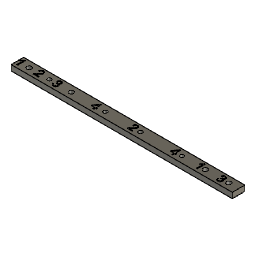
Base Board Tester v1 (Autodesk Fusion 360 design; units mm, degrees)
Autodesk Fusion 360 part; units mm, degrees
sketch "Sketch1" plane through (0, 0, 0) normal (0, 0, 1) x (1, 0, 0)
  line L0 (-51.9584, -20.427) -> (88.8166, -20.427)
  line L1 (88.8166, -20.427) -> (88.8166, -28.427)
  line L2 (88.8166, -28.427) -> (-51.9584, -28.427)
  line L3 (-51.9584, -28.427) -> (-51.9584, -20.427)
  circle A0 centre (-17.6214, -24.427) radius 1.5
  circle A1 centre (82.5086, -24.427) radius 1.5
  circle A2 centre (-44.4942, -24.427) radius 1.5
  circle A3 centre (67.7058, -24.427) radius 1.5
  circle A4 centre (4, -24.427) radius 1.25
  circle A5 centre (52.78, -24.427) radius 1.25
  circle A6 centre (-31.6334, -24.427) radius 1.25
  circle A7 centre (26.3666, -24.427) radius 1.25
  line L4 (-49.5707, -26.5817) -> (-50.1846, -26.5817)
  line L5 (-50.1846, -26.5817) -> (-50.1846, -22.6697)
  spline S0 degree 2 poles (-50.1846, -22.6697) (-50.4063, -22.8811) (-50.7679, -23.0926) knots 0 0 0 1 1 1
  spline S1 degree 2 poles (-50.7679, -23.0926) (-51.126, -23.304) (-51.4125, -23.4098) knots 0 0 0 1 1 1
  line L6 (-51.4125, -23.4098) -> (-51.4125, -22.8163)
  spline S2 degree 2 poles (-51.4125, -22.8163) (-50.8975, -22.5742) (-50.5121, -22.2297) knots 0 0 0 1 1 1
  spline S3 degree 2 poles (-50.5121, -22.2297) (-50.1267, -21.8852) (-49.9664, -21.5612) knots 0 0 0 1 1 1
  line L7 (-49.9664, -21.5612) -> (-49.5707, -21.5612)
  line L8 (-49.5707, -21.5612) -> (-49.5707, -26.5817)
  line L9 (-36.5983, -26.0261) -> (-36.5983, -26.6161)
  line L10 (-36.5983, -26.6161) -> (-39.9033, -26.6161)
  spline S4 degree 2 poles (-39.9033, -26.6161) (-39.9101, -26.3944) (-39.8316, -26.1898) knots 0 0 0 1 1 1
  spline S5 degree 2 poles (-39.8316, -26.1898) (-39.7054, -25.8521) (-39.4292, -25.5247) knots 0 0 0 1 1 1
  spline S6 degree 2 poles (-39.4292, -25.5247) (-39.1495, -25.1973) (-38.6243, -24.7675) knots 0 0 0 1 1 1
  spline S7 degree 2 poles (-38.6243, -24.7675) (-37.8091, -24.0991) (-37.5226, -23.7102) knots 0 0 0 1 1 1
  spline S8 degree 2 poles (-37.5226, -23.7102) (-37.2361, -23.318) (-37.2361, -22.9701) knots 0 0 0 1 1 1
  spline S9 degree 2 poles (-37.2361, -22.9701) (-37.2361, -22.6052) (-37.4988, -22.3562) knots 0 0 0 1 1 1
  spline S10 degree 2 poles (-37.4988, -22.3562) (-37.758, -22.1038) (-38.1775, -22.1038) knots 0 0 0 1 1 1
  spline S11 degree 2 poles (-38.1775, -22.1038) (-38.6209, -22.1038) (-38.8869, -22.3699) knots 0 0 0 1 1 1
  spline S12 degree 2 poles (-38.8869, -22.3699) (-39.1529, -22.6359) (-39.1563, -23.1066) knots 0 0 0 1 1 1
  line L11 (-39.1563, -23.1066) -> (-39.7873, -23.0418)
  spline S13 degree 2 poles (-39.7873, -23.0418) (-39.7225, -22.3358) (-39.2996, -21.9674) knots 0 0 0 1 1 1
  spline S14 degree 2 poles (-39.2996, -21.9674) (-38.8767, -21.5957) (-38.1638, -21.5957) knots 0 0 0 1 1 1
  spline S15 degree 2 poles (-38.1638, -21.5957) (-37.4442, -21.5957) (-37.0247, -21.9947) knots 0 0 0 1 1 1
  spline S16 degree 2 poles (-37.0247, -21.9947) (-36.6052, -22.3937) (-36.6052, -22.9838) knots 0 0 0 1 1 1
  spline S17 degree 2 poles (-36.6052, -22.9838) (-36.6052, -23.2839) (-36.7279, -23.5738) knots 0 0 0 1 1 1
  spline S18 degree 2 poles (-36.7279, -23.5738) (-36.8507, -23.8637) (-37.1372, -24.1843) knots 0 0 0 1 1 1
  spline S19 degree 2 poles (-37.1372, -24.1843) (-37.4203, -24.5049) (-38.082, -25.0643) knots 0 0 0 1 1 1
  spline S20 degree 2 poles (-38.082, -25.0643) (-38.6345, -25.5281) (-38.7914, -25.6952) knots 0 0 0 1 1 1
  spline S21 degree 2 poles (-38.7914, -25.6952) (-38.9483, -25.859) (-39.0506, -26.0261) knots 0 0 0 1 1 1
  line L12 (-39.0506, -26.0261) -> (-36.5983, -26.0261)
  line L13 (-28.4362, -25.3635) -> (-27.8223, -25.2816)
  spline S22 degree 2 poles (-27.8223, -25.2816) (-27.7166, -25.8035) (-27.4642, -26.0354) knots 0 0 0 1 1 1
  spline S23 degree 2 poles (-27.4642, -26.0354) (-27.2084, -26.2639) (-26.8435, -26.2639) knots 0 0 0 1 1 1
  spline S24 degree 2 poles (-26.8435, -26.2639) (-26.4103, -26.2639) (-26.1136, -25.9638) knots 0 0 0 1 1 1
  spline S25 degree 2 poles (-26.1136, -25.9638) (-25.8134, -25.6636) (-25.8134, -25.2203) knots 0 0 0 1 1 1
  spline S26 degree 2 poles (-25.8134, -25.2203) (-25.8134, -24.7973) (-26.0897, -24.5245) knots 0 0 0 1 1 1
  spline S27 degree 2 poles (-26.0897, -24.5245) (-26.366, -24.2482) (-26.7923, -24.2482) knots 0 0 0 1 1 1
  spline S28 degree 2 poles (-26.7923, -24.2482) (-26.9662, -24.2482) (-27.2254, -24.3164) knots 0 0 0 1 1 1
  line L14 (-27.2254, -24.3164) -> (-27.1572, -23.7776)
  spline S29 degree 2 poles (-27.1572, -23.7776) (-27.0958, -23.7844) (-27.0583, -23.7844) knots 0 0 0 1 1 1
  spline S30 degree 2 poles (-27.0583, -23.7844) (-26.6661, -23.7844) (-26.3523, -23.5797) knots 0 0 0 1 1 1
  spline S31 degree 2 poles (-26.3523, -23.5797) (-26.0385, -23.3751) (-26.0385, -22.9488) knots 0 0 0 1 1 1
  spline S32 degree 2 poles (-26.0385, -22.9488) (-26.0385, -22.6111) (-26.2671, -22.3894) knots 0 0 0 1 1 1
  spline S33 degree 2 poles (-26.2671, -22.3894) (-26.4956, -22.1677) (-26.8571, -22.1677) knots 0 0 0 1 1 1
  spline S34 degree 2 poles (-26.8571, -22.1677) (-27.2152, -22.1677) (-27.454, -22.3928) knots 0 0 0 1 1 1
  spline S35 degree 2 poles (-27.454, -22.3928) (-27.6927, -22.6179) (-27.7609, -23.0681) knots 0 0 0 1 1 1
  line L15 (-27.7609, -23.0681) -> (-28.3748, -22.959)
  spline S36 degree 2 poles (-28.3748, -22.959) (-28.2623, -22.3417) (-27.8632, -22.004) knots 0 0 0 1 1 1
  spline S37 degree 2 poles (-27.8632, -22.004) (-27.4642, -21.663) (-26.8707, -21.663) knots 0 0 0 1 1 1
  spline S38 degree 2 poles (-26.8707, -21.663) (-26.4615, -21.663) (-26.117, -21.8403) knots 0 0 0 1 1 1
  spline S39 degree 2 poles (-26.117, -21.8403) (-25.7725, -22.0143) (-25.5918, -22.3178) knots 0 0 0 1 1 1
  spline S40 degree 2 poles (-25.5918, -22.3178) (-25.4076, -22.6213) (-25.4076, -22.9624) knots 0 0 0 1 1 1
  spline S41 degree 2 poles (-25.4076, -22.9624) (-25.4076, -23.2864) (-25.5815, -23.5525) knots 0 0 0 1 1 1
  spline S42 degree 2 poles (-25.5815, -23.5525) (-25.7555, -23.8185) (-26.0965, -23.9754) knots 0 0 0 1 1 1
  spline S43 degree 2 poles (-26.0965, -23.9754) (-25.6531, -24.0777) (-25.4076, -24.4017) knots 0 0 0 1 1 1
  spline S44 degree 2 poles (-25.4076, -24.4017) (-25.162, -24.7223) (-25.162, -25.2066) knots 0 0 0 1 1 1
  spline S45 degree 2 poles (-25.162, -25.2066) (-25.162, -25.8615) (-25.6395, -26.3185) knots 0 0 0 1 1 1
  spline S46 degree 2 poles (-25.6395, -26.3185) (-26.117, -26.7721) (-26.8469, -26.7721) knots 0 0 0 1 1 1
  spline S47 degree 2 poles (-26.8469, -26.7721) (-27.5051, -26.7721) (-27.9417, -26.3799) knots 0 0 0 1 1 1
  spline S48 degree 2 poles (-27.9417, -26.3799) (-28.3748, -25.9877) (-28.4362, -25.3635) knots 0 0 0 1 1 1
  line L16 (-1.7271, -26.6568) -> (-1.7271, -25.4597)
  line L17 (-1.7271, -25.4597) -> (-3.8963, -25.4597)
  line L18 (-3.8963, -25.4597) -> (-3.8963, -24.8969)
  line L19 (-3.8963, -24.8969) -> (-1.6146, -21.6568)
  line L20 (-1.6146, -21.6568) -> (-1.1132, -21.6568)
  line L21 (-1.1132, -21.6568) -> (-1.1132, -24.8969)
  line L22 (-1.1132, -24.8969) -> (-0.4379, -24.8969)
  line L23 (-0.4379, -24.8969) -> (-0.4379, -25.4597)
  line L24 (-0.4379, -25.4597) -> (-1.1132, -25.4597)
  line L25 (-1.1132, -25.4597) -> (-1.1132, -26.6568)
  line L26 (-1.1132, -26.6568) -> (-1.7271, -26.6568)
  line L27 (-1.7271, -24.8969) -> (-1.7271, -22.6425)
  line L28 (-1.7271, -22.6425) -> (-3.2926, -24.8969)
  line L29 (-3.2926, -24.8969) -> (-1.7271, -24.8969)
  line L30 (23.274, -25.9995) -> (23.274, -26.5895)
  line L31 (23.274, -26.5895) -> (19.9691, -26.5895)
  spline S49 degree 2 poles (19.9691, -26.5895) (19.9623, -26.3678) (20.0408, -26.1632) knots 0 0 0 1 1 1
  spline S50 degree 2 poles (20.0408, -26.1632) (20.1669, -25.8255) (20.4432, -25.4981) knots 0 0 0 1 1 1
  spline S51 degree 2 poles (20.4432, -25.4981) (20.7229, -25.1707) (21.2481, -24.7409) knots 0 0 0 1 1 1
  spline S52 degree 2 poles (21.2481, -24.7409) (22.0633, -24.0725) (22.3498, -23.6836) knots 0 0 0 1 1 1
  spline S53 degree 2 poles (22.3498, -23.6836) (22.6363, -23.2914) (22.6363, -22.9435) knots 0 0 0 1 1 1
  spline S54 degree 2 poles (22.6363, -22.9435) (22.6363, -22.5786) (22.3736, -22.3296) knots 0 0 0 1 1 1
  spline S55 degree 2 poles (22.3736, -22.3296) (22.1144, -22.0772) (21.6949, -22.0772) knots 0 0 0 1 1 1
  spline S56 degree 2 poles (21.6949, -22.0772) (21.2515, -22.0772) (20.9855, -22.3433) knots 0 0 0 1 1 1
  spline S57 degree 2 poles (20.9855, -22.3433) (20.7195, -22.6093) (20.7161, -23.08) knots 0 0 0 1 1 1
  line L32 (20.7161, -23.08) -> (20.0851, -23.0152)
  spline S58 degree 2 poles (20.0851, -23.0152) (20.1499, -22.3092) (20.5728, -21.9408) knots 0 0 0 1 1 1
  spline S59 degree 2 poles (20.5728, -21.9408) (20.9957, -21.5691) (21.7086, -21.5691) knots 0 0 0 1 1 1
  spline S60 degree 2 poles (21.7086, -21.5691) (22.4282, -21.5691) (22.8477, -21.9681) knots 0 0 0 1 1 1
  spline S61 degree 2 poles (22.8477, -21.9681) (23.2672, -22.3671) (23.2672, -22.9572) knots 0 0 0 1 1 1
  spline S62 degree 2 poles (23.2672, -22.9572) (23.2672, -23.2573) (23.1444, -23.5472) knots 0 0 0 1 1 1
  spline S63 degree 2 poles (23.1444, -23.5472) (23.0217, -23.8371) (22.7352, -24.1577) knots 0 0 0 1 1 1
  spline S64 degree 2 poles (22.7352, -24.1577) (22.4521, -24.4783) (21.7904, -25.0377) knots 0 0 0 1 1 1
  spline S65 degree 2 poles (21.7904, -25.0377) (21.2379, -25.5015) (21.081, -25.6686) knots 0 0 0 1 1 1
  spline S66 degree 2 poles (21.081, -25.6686) (20.9241, -25.8324) (20.8218, -25.9995) knots 0 0 0 1 1 1
  line L33 (20.8218, -25.9995) -> (23.274, -25.9995)
  line L34 (48.5734, -26.6302) -> (48.5734, -25.4331)
  line L35 (48.5734, -25.4331) -> (46.4043, -25.4331)
  line L36 (46.4043, -25.4331) -> (46.4043, -24.8703)
  line L37 (46.4043, -24.8703) -> (48.686, -21.6302)
  line L38 (48.686, -21.6302) -> (49.1874, -21.6302)
  line L39 (49.1874, -21.6302) -> (49.1874, -24.8703)
  line L40 (49.1874, -24.8703) -> (49.8627, -24.8703)
  line L41 (49.8627, -24.8703) -> (49.8627, -25.4331)
  line L42 (49.8627, -25.4331) -> (49.1874, -25.4331)
  line L43 (49.1874, -25.4331) -> (49.1874, -26.6302)
  line L44 (49.1874, -26.6302) -> (48.5734, -26.6302)
  line L45 (48.5734, -24.8703) -> (48.5734, -22.6159)
  line L46 (48.5734, -22.6159) -> (47.008, -24.8703)
  line L47 (47.008, -24.8703) -> (48.5734, -24.8703)
  line L48 (64.694, -26.5401) -> (64.0801, -26.5401)
  line L49 (64.0801, -26.5401) -> (64.0801, -22.6281)
  spline S67 degree 2 poles (64.0801, -22.6281) (63.8584, -22.8396) (63.4969, -23.0511) knots 0 0 0 1 1 1
  spline S68 degree 2 poles (63.4969, -23.0511) (63.1388, -23.2625) (62.8523, -23.3683) knots 0 0 0 1 1 1
  line L50 (62.8523, -23.3683) -> (62.8523, -22.7748)
  spline S69 degree 2 poles (62.8523, -22.7748) (63.3673, -22.5326) (63.7527, -22.1882) knots 0 0 0 1 1 1
  spline S70 degree 2 poles (63.7527, -22.1882) (64.1381, -21.8437) (64.2984, -21.5197) knots 0 0 0 1 1 1
  line L51 (64.2984, -21.5197) -> (64.694, -21.5197)
  line L52 (64.694, -21.5197) -> (64.694, -26.5401)
  line L53 (76.3325, -25.4509) -> (76.9464, -25.369)
  spline S71 degree 2 poles (76.9464, -25.369) (77.0521, -25.8908) (77.3045, -26.1228) knots 0 0 0 1 1 1
  spline S72 degree 2 poles (77.3045, -26.1228) (77.5603, -26.3513) (77.9253, -26.3513) knots 0 0 0 1 1 1
  spline S73 degree 2 poles (77.9253, -26.3513) (78.3584, -26.3513) (78.6551, -26.0511) knots 0 0 0 1 1 1
  spline S74 degree 2 poles (78.6551, -26.0511) (78.9553, -25.751) (78.9553, -25.3076) knots 0 0 0 1 1 1
  spline S75 degree 2 poles (78.9553, -25.3076) (78.9553, -24.8847) (78.679, -24.6118) knots 0 0 0 1 1 1
  spline S76 degree 2 poles (78.679, -24.6118) (78.4027, -24.3356) (77.9764, -24.3356) knots 0 0 0 1 1 1
  spline S77 degree 2 poles (77.9764, -24.3356) (77.8025, -24.3356) (77.5433, -24.4038) knots 0 0 0 1 1 1
  line L54 (77.5433, -24.4038) -> (77.6115, -23.8649)
  spline S78 degree 2 poles (77.6115, -23.8649) (77.6729, -23.8717) (77.7104, -23.8717) knots 0 0 0 1 1 1
  spline S79 degree 2 poles (77.7104, -23.8717) (78.1026, -23.8717) (78.4164, -23.6671) knots 0 0 0 1 1 1
  spline S80 degree 2 poles (78.4164, -23.6671) (78.7302, -23.4625) (78.7302, -23.0361) knots 0 0 0 1 1 1
  spline S81 degree 2 poles (78.7302, -23.0361) (78.7302, -22.6985) (78.5017, -22.4768) knots 0 0 0 1 1 1
  spline S82 degree 2 poles (78.5017, -22.4768) (78.2731, -22.2551) (77.9116, -22.2551) knots 0 0 0 1 1 1
  spline S83 degree 2 poles (77.9116, -22.2551) (77.5535, -22.2551) (77.3148, -22.4802) knots 0 0 0 1 1 1
  spline S84 degree 2 poles (77.3148, -22.4802) (77.076, -22.7053) (77.0078, -23.1555) knots 0 0 0 1 1 1
  line L55 (77.0078, -23.1555) -> (76.3939, -23.0464)
  spline S85 degree 2 poles (76.3939, -23.0464) (76.5064, -22.429) (76.9055, -22.0914) knots 0 0 0 1 1 1
  spline S86 degree 2 poles (76.9055, -22.0914) (77.3045, -21.7503) (77.898, -21.7503) knots 0 0 0 1 1 1
  spline S87 degree 2 poles (77.898, -21.7503) (78.3073, -21.7503) (78.6517, -21.9277) knots 0 0 0 1 1 1
  spline S88 degree 2 poles (78.6517, -21.9277) (78.9962, -22.1016) (79.177, -22.4052) knots 0 0 0 1 1 1
  spline S89 degree 2 poles (79.177, -22.4052) (79.3611, -22.7087) (79.3611, -23.0498) knots 0 0 0 1 1 1
  spline S90 degree 2 poles (79.3611, -23.0498) (79.3611, -23.3738) (79.1872, -23.6398) knots 0 0 0 1 1 1
  spline S91 degree 2 poles (79.1872, -23.6398) (79.0133, -23.9058) (78.6722, -24.0627) knots 0 0 0 1 1 1
  spline S92 degree 2 poles (78.6722, -24.0627) (79.1156, -24.165) (79.3611, -24.4891) knots 0 0 0 1 1 1
  spline S93 degree 2 poles (79.3611, -24.4891) (79.6067, -24.8097) (79.6067, -25.294) knots 0 0 0 1 1 1
  spline S94 degree 2 poles (79.6067, -25.294) (79.6067, -25.9488) (79.1292, -26.4058) knots 0 0 0 1 1 1
  spline S95 degree 2 poles (79.1292, -26.4058) (78.6517, -26.8594) (77.9218, -26.8594) knots 0 0 0 1 1 1
  spline S96 degree 2 poles (77.9218, -26.8594) (77.2636, -26.8594) (76.827, -26.4672) knots 0 0 0 1 1 1
  spline S97 degree 2 poles (76.827, -26.4672) (76.3939, -26.075) (76.3325, -25.4509) knots 0 0 0 1 1 1
  dimension "d2" = 3
  dimension "d3" = 3
  dimension "d4" = 100.13
  dimension "d6" = 8
  dimension "d7" = 3
  dimension "d8" = 3
  dimension "d9" = 112.2
  dimension "d11" = 4
  dimension "d12" = 4
  dimension "d14" = 2.5
  dimension "d15" = 2.5
  dimension "d18" = 4
  dimension "d20" = 4
  dimension "d27" = 48.78
  dimension "d28" = 2.5
  dimension "d29" = 2.5
  dimension "d30" = 58
  dimension "d31" = 4
  dimension "d46" = 4
  dimension "d47" = 4
  dimension "d48" = 4
  constraint horizontal L0
  constraint vertical L1
  constraint horizontal L2
  constraint vertical L3
  measures "d2" diameter of A0
  measures "d3" diameter of A1
  measures "d4" distance of A0.centre A1.centre
  measures "d6" distance of L0.start L2.end
  measures "d7" diameter of A2
  measures "d8" diameter of A3
  measures "d9" distance of A2.centre A3.centre
  measures "d11" distance of L0 A2.centre
  measures "d12" distance of L0 A0.centre
  measures "d14" diameter of A4
  measures "d15" diameter of A5
  measures "d18" distance of L0 A4.centre
  measures "d20" distance of L0 A5.centre
  measures "d27" distance of A4.centre A5.centre
  measures "d28" diameter of A6
  measures "d29" diameter of A7
  measures "d30" horizontal distance of A6.centre A7.centre
  measures "d31" distance of L0 A6.centre
  measures "d46" distance of L0 A7.centre
  measures "d47" distance of L0 A3.centre
  measures "d48" distance of L0 A1.centre
extrude "Extrude3" add sketch "Sketch1" along normal blind 3.5 contours L0 L1 L2 L3 | L4 L5 S0 S1 L6 S2 S3 L7 L8 | L9 L10 S4 S5 S6 S7 S8 S9 S10 S11 S12 L11 S13 S14 S15 S16 S17 S18 S19 S20 S21 L12 | L13 S22 S23 S24 S25 S26 S27 S28 L14 S29 S30 S31 S32 S33 S34 S35 L15 S36 S37 S38 S39 S40 S41 S42 S43 S44 S45 S46 S47 S48 | L16 L17 L18 L19 L20 L21 L22 L23 L24 L25 L26 | L27 L28 L29 | L30 L31 S49 S50 S51 S52 S53 S54 S55 S56 S57 L32 S58 S59 S60 S61 S62 S63 S64 S65 S66 L33 | L34 L35 L36 L37 L38 L39 L40 L41 L42 L43 L44 | L45 L46 L47 | L48 L49 S67 S68 L50 S69 S70 L51 L52 | L53 S71 S72 S73 S74 S75 S76 S77 L54 S78 S79 S80 S81 S82 S83 S84 L55 S85 S86 S87 S88 S89 S90 S91 S92 S93 S94 S95 S96 S97
split_face "SplitFace1" 1 faces at (-49.9703, -24.427, 3.5) by curves path "Sketch1" along L6 S2 S3 L7 L8 L4 L5 S0 S1
split_face "SplitFace2" 1 faces at (87.2139, -24.427, 3.5) by curves path "Sketch1" along S19 S20 S21 L12 L9 L10 S4 S5 S6 S7 S8 S9 S10 S11 S12 L11 S13 S14 S15 S16 S17 S18
split_face "SplitFace3" 1 faces at (87.2139, -24.427, 3.5) by curves path "Sketch1" along S45 S46 S47 S48 L13 S22 S23 S24 S25 S26 S27 S28 L14 S29 S30 S31 S32 S33 S34 S35 L15 S36 S37 S38 S39 S40 S41 S42 S43 S44
split_face "SplitFace4" 1 faces at (87.2139, -24.427, 3.5) by curves path "Sketch1" along L23 L24 L25 L26 L16 L17 L18 L19 L20 L21 L22
split_face "SplitFace5" 1 faces at (87.2139, -24.427, 3.5) by curves path "Sketch1" along S54 S55 S56 S57 L32 S58 S59 S60 S61 S62 S63 S64 S65 S66 L33 L30 L31 S49 S50 S51 S52 S53
split_face "SplitFace6" 1 faces at (87.2139, -24.427, 3.5) by curves path "Sketch1" along L41 L42 L43 L44 L34 L35 L36 L37 L38 L39 L40
split_face "SplitFace7" 1 faces at (87.2139, -24.427, 3.5) by curves path "Sketch1" along L50 S69 S70 L51 L52 L48 L49 S67 S68
split_face "SplitFace8" 1 faces at (87.2139, -24.427, 3.5) by curves path "Sketch1" along S93 S94 S95 S96 S97 L53 S71 S72 S73 S74 S75 S76 S77 L54 S78 S79 S80 S81 S82 S83 S84 L55 S85 S86 S87 S88 S89 S90 S91 S92
move_face "OffsetFaces1" offset -0.5 8 faces at (-49.7754, -23.6042, 3.5) (-38.5174, -26.4194, 3.5) (-26.381, -23.9731, 3.5) (-2.208, -23.8169, 3.5) (21.355, -26.3928, 3.5) (48.0925, -23.7903, 3.5) (64.4894, -23.5627, 3.5) (78.3878, -24.0605, 3.5)
